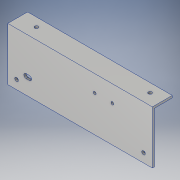
# Autodesk Inventor part: CAR_019_TensionerLBracket
Saved by Autodesk Inventor 2018 (Build 220112000, 112)
## iProperties
Created: 2020-02-01
Part Number: CAR_019_TensionerLBracket
Material: Aluminum 6061
Document SubType Name: Modeling
Designer: user
Density: 2.7 g/cm^3
Appearance: Aluminum - Flat
Mass: 112.115 g
Surface Area: 284.947 cm^2
Volume: 41.5242 cm^3
Author: user
Autodesk Inventor part; units mm, degrees
ref_plane "YZ Plane" through (0, 0, 0) normal (1, 0, 0) x (0, 1, 0)
ref_plane "XZ Plane" through (0, 0, 0) normal (0, 1, 0) x (-1, 0, 0)
ref_plane "XY Plane" through (0, 0, 0) normal (0, 0, 1) x (1, 0, 0)
sketch "Sketch1" plane through (0, 0, 0) normal (1, 0, 0) x (0, 1, 0)
  line L0 (0, 0) -> (76.2, 0)
  line L1 (76.2, 0) -> (76.2, -3.175)
  line L2 (76.2, -3.175) -> (0, -3.175)
  line L3 (0, -3.175) -> (0, 0)
  line L4 (76.2, 0) -> (73.025, 0)
  line L5 (73.025, 0) -> (73.025, -28.575)
  line L6 (73.025, -28.575) -> (76.2, -28.575)
  line L7 (76.2, -28.575) -> (76.2, 0)
  dimension "d0" = 76.2
  dimension "d1" = 3.175
  dimension "d2" = 28.575
  constraints: 16 end point, 4 parallel, 3 perpendicular, 2 horizontal
  measures "d0" distance of L0.start L0.end
  measures "d1" distance of L2.end L0.start
  measures "d2" distance of L6.end L0.end
extrude "Extrusion1" add sketch "Sketch1" along normal blind 207.9244
sketch "Sketch2" plane through (0, 0, -3.175) normal (0, 0, -1) x (-1, 0, 0)
  line L0 (-207.9244, 0) -> (-207.9244, 73.025) projected
  line L1 (0, 76.2) -> (-207.9244, 76.2) projected
  point P0 (0, 0)
  point P1 (-150.4442, 51.9938)
  point P2 (-125.0442, 51.9938)
  dimension "d5" = 57.4802
  dimension "d6" = 82.8802
  dimension "d7" = 24.2062
  dimension "d8" = 24.2062
  measures "d5" distance from line of L0 point (-150.444, 51.994)
  measures "d6" distance from line of L0 point (-125.044, 51.994)
  measures "d7" distance from line of L1 point (-125.044, 51.994)
  measures "d8" distance from line of L1 point (-150.444, 51.994)
hole "Hole1" at (150.4442, 51.9938, -3.175) at (125.0442, 51.9938, -3.175) direction (0, 0, 1) diameter 4.0386 end through all
sketch "Sketch5" plane through (0, 76.2, 0) normal (0, 1, 0) x (1, 0, 0)
  line L0 (0, 28.575) -> (207.9244, 28.575) projected
  line L1 (207.9244, 28.575) -> (207.9244, 0) projected
  line L2 (0, 28.575) -> (0, 0) projected
  point P0 (188.8744, 15.875)
  point P1 (25.4, 15.875)
  dimension "d43" = 12.7
  dimension "d44" = 12.7
  dimension "d45" = 19.05
  dimension "d46" = 25.4
  measures "d43" distance from line of L0 point (188.874, 15.875)
  measures "d44" distance from line of L0 point (25.4, 15.875)
  measures "d45" distance from line of L1 point (188.874, 15.875)
  measures "d46" distance from line of L2 point (25.4, 15.875)
sketch "Sketch6" plane through (0, 0, -3.175) normal (0, 0, -1) x (-1, 0, 0)
  line L0 (0, 0) -> (-207.9244, 0) projected
  line L1 (-207.9244, 0) -> (-207.9244, 73.025) projected
  line L2 (0, 0) -> (0, 73.025) projected
  point P0 (-195.2244, 12.7)
  point P1 (-12.7, 12.7)
  dimension "d47" = 12.7
  dimension "d48" = 12.7
  dimension "d49" = 12.7
  dimension "d50" = 12.7
  measures "d47" distance from line of L0 point (-195.224, 12.7)
  measures "d48" distance from line of L1 point (-195.224, 12.7)
  measures "d49" distance from line of L0 point (-12.7, 12.7)
  measures "d50" distance from line of point (-12.7, 12.7) L2
hole "Hole4" at (195.2244, 12.7, -3.175) at (12.7, 12.7, -3.175) direction (0, 0, 1) diameter 5.1054 end through all clearance for "Flat Head Machine Screw (82)" size "#10" standard "Ansi Unified Screw Threads"
hole "Hole3" at (25.4, 76.2, -15.875) at (188.8744, 76.2, -15.875) direction (0, -1, 0) diameter 5.1054 end through all clearance for "Flat Head Machine Screw (82)" size "#10" standard "Ansi Unified Screw Threads"
sketch "Sketch7" plane through (0, 0, 0) normal (0, 0, 1) x (1, 0, 0)
  line L0 (0, 0) -> (207.9244, 0) projected
  line L1 (207.9244, 76.2) -> (207.9244, 0) projected
  line L2 (0, 76.2) -> (0, 0) projected
  point P0 (26.3398, 23.7998)
  dimension "d67" = 23.7998
  dimension "d76" = 26.3398
  measures "d67" distance from line of L0 point (26.34, 23.8)
  measures "d76" distance from line of L2 point (26.34, 23.8)
hole "Hole5" at (26.3398, 23.7998, 0) direction (0, 0, -1) diameter 6.35 end through all
sketch "Sketch8" plane through (0, 0, 0) normal (0, 0, 1) x (1, 0, 0)
  circle A0 centre (26.3398, 23.7998) radius 3.175 projected
  line L0 (26.3398, 23.7998) -> (31.1023, 23.7998) construction
  line L1 (26.3398, 20.6248) -> (31.1023, 20.6248)
  line L2 (31.1023, 26.9748) -> (26.3398, 26.9748)
  arc A1 (26.3398, 26.9748) -> (26.3398, 20.6248) centre (26.3398, 23.7998) ccw
  arc A2 (31.1023, 20.6248) -> (31.1023, 26.9748) centre (31.1023, 23.7998) ccw
  point P0 (0, 0)
  point P1 (28.721, 23.7998)
  dimension "d77" = 4.7625
  constraints: 8 end point, 4 point on circle, 4 tangent, 2 centre point, 1 concentric, 1 horizontal, 1 midpoint, 1 parallel
  measures "d77" distance of L0.start L0.end
extrude "Extrusion3" cut sketch "Sketch8" against normal blind 25.4 contours A0 L2 A2 L1
sketch "Sketch3" plane through (0, 0, -3.175) normal (0, 0, -1) x (-1, 0, 0)
  line L0 (-158.5408, 14.5542) -> (38.7343, 14.5542) construction
  line L1 (0, 76.2) -> (-207.9244, 76.2) construction
  line L2 (-161.6607, 44.1198) -> (30.0945, 44.1198) construction
  line L3 (-31.75, 37.7698) -> (-12.7, 37.7698) construction
  line L4 (-31.75, 35.2806) -> (-12.7, 35.2806)
  line L5 (-12.7, 40.259) -> (-31.75, 40.259)
  arc A0 (-31.75, 40.259) -> (-31.75, 35.2806) centre (-31.75, 37.7698) ccw
  arc A1 (-12.7, 35.2806) -> (-12.7, 40.259) centre (-12.7, 37.7698) ccw
  line L6 (-31.75, 25.4) -> (-12.7, 25.4) construction
  line L7 (-31.75, 22.9108) -> (-12.7, 22.9108)
  line L8 (-12.7, 27.8892) -> (-31.75, 27.8892)
  arc A2 (-31.75, 27.8892) -> (-31.75, 22.9108) centre (-31.75, 25.4) ccw
  arc A3 (-12.7, 22.9108) -> (-12.7, 27.8892) centre (-12.7, 25.4) ccw
  line L9 (0, 0) -> (0, 73.025) projected
  line L10 (-69.85, 37.7698) -> (-50.8, 37.7698) construction
  line L11 (-69.85, 35.2806) -> (-50.8, 35.2806)
  line L12 (-50.8, 40.259) -> (-69.85, 40.259)
  arc A4 (-69.85, 40.259) -> (-69.85, 35.2806) centre (-69.85, 37.7698) ccw
  arc A5 (-50.8, 35.2806) -> (-50.8, 40.259) centre (-50.8, 37.7698) ccw
  point P0 (-22.225, 37.7698)
  point P1 (-22.225, 25.4)
  point P2 (-60.325, 37.7698)
  dimension "d16" = 61.6458
  dimension "d17" = 29.5656
  dimension "d19" = 2.4892
  dimension "d20" = 6.35
  dimension "d29" = 38.1
  dimension "d30" = 6.35
  dimension "d31" = 19.05
  dimension "d32" = 31.75
  dimension "d33" = 31.75
  dimension "d65" = 10.8458
  constraints: 28 end point, 12 point on circle, 12 tangent, 6 centre point, 4 horizontal, 4 parallel, 3 midpoint, 2 equal length, 2 equal radius
  measures "d16" distance between parallel lines of L1 L0
  measures "d17" distance between parallel lines of L0 L2
  measures "d19" radius of A3
  measures "d20" distance between parallel lines of L2 L3
  measures "d29" distance of L3.start L10.start
  measures "d30" distance between parallel lines of L10 L2
  measures "d31" distance of L6.start L6.end
  measures "d32" distance from line of L9 L6.start
  measures "d33" distance from line of L9 L3.start
  measures "d65" distance between parallel lines of L0 L6
sketch "Sketch4" plane through (0, 0, -3.175) normal (0, 0, -1) x (-1, 0, 0)
  line L0 (-12.7, 35.2806) -> (-31.75, 35.2806) projected
  arc A0 (-12.7, 22.9108) -> (-12.7, 27.8892) centre (-12.7, 25.4) ccw projected
  line L1 (-12.7, 22.9108) -> (-31.75, 22.9108) projected
  arc A1 (-31.75, 27.8892) -> (-31.75, 22.9108) centre (-31.75, 25.4) ccw projected
  line L2 (-31.75, 27.8892) -> (-12.7, 27.8892) projected
  arc A2 (-12.7, 35.2806) -> (-12.7, 40.259) centre (-12.7, 37.7698) ccw projected
  line L3 (-12.7, 35.2806) -> (-31.75, 35.2806) projected
  arc A3 (-31.75, 40.259) -> (-31.75, 35.2806) centre (-31.75, 37.7698) ccw projected
  line L4 (-31.75, 40.259) -> (-12.7, 40.259) projected
  arc A4 (-50.8, 35.2806) -> (-50.8, 40.259) centre (-50.8, 37.7698) ccw projected
  line L5 (-50.8, 35.2806) -> (-69.85, 35.2806) projected
  arc A5 (-69.85, 40.259) -> (-69.85, 35.2806) centre (-69.85, 37.7698) ccw projected
  line L6 (-69.85, 40.259) -> (-50.8, 40.259) projected
  circle A6 centre (-125.0442, 51.9938) radius 2.0193 projected
  circle A7 centre (-99.6442, 51.9938) radius 2.0193 projected
  line L7 (-182.5244, 73.025) -> (0, 73.025) projected
  line L8 (-182.5244, 0) -> (-182.5244, 73.025) projected
  line L9 (0, 0) -> (-182.5244, 0) projected
  line L10 (0, 0) -> (0, 73.025) projected
  point P0 (0, 0)
  point P1 (-9.652, 31.5849)
  dimension "d34" = 3.6957
  dimension "d35" = 22.098
  dimension "d66" = 7.3914
  measures "d34" distance from line of L0 point (-9.652, 31.585)
  measures "d35" horizontal distance of A3.centre point (-9.652, 31.585)
  measures "d66" distance between parallel lines of L2 L0
equation "\"d8\" = d7"
equation "\"d30\" = d20"
equation "\"d33\" = d32"
equation "\"d34\" = 0.5 * d66"
body "Solid1"
